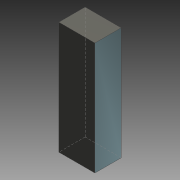
# Autodesk Inventor part: Battery - 3S 2200mAh
Saved by Autodesk Inventor 2012 (Build 160160000, 160)
## iProperties
Created: 2013-03-14
Part Number: Battery - 3S 2200mAh
Material: Default
Document SubType Name: Modeling
Designer: fixer
Mass: 175 g
Surface Area: 139.807 cm^2
Volume: 87.7349 cm^3
Density: 1.99464 g/cm^3
Author: fixer
Autodesk Inventor part; units mm, degrees
ref_plane "YZ Plane" through (0, 0, 0) normal (1, 0, 0) x (0, 1, 0)
ref_plane "XZ Plane" through (0, 0, 0) normal (0, 1, 0) x (-1, 0, 0)
ref_plane "XY Plane" through (0, 0, 0) normal (0, 0, 1) x (1, 0, 0)
sketch "Sketch1" plane through (0, 0, 0) normal (0, 0, 1) x (1, 0, 0)
  line L0 (16.891, -52.705) -> (-16.891, -52.705)
  line L1 (-16.891, -52.705) -> (-16.891, 52.705)
  line L2 (-16.891, 52.705) -> (16.891, 52.705)
  line L3 (16.891, 52.705) -> (16.891, -52.705)
  point P0 (0, 0)
  point P1 (-16.891, 0)
  point P2 (0, 52.705)
  dimension "d0" = 105.41
  dimension "d1" = 33.782
  constraints: 8 end point, 2 midpoint, 2 parallel, 1 horizontal, 1 horizontal alignment, 1 perpendicular, 1 vertical alignment
  measures "d0" distance of L0.end L1.end
  measures "d1" distance of L0.start L0.end
extrude "Extrusion1" add sketch "Sketch1" along normal blind 24.638
body "Solid1"
